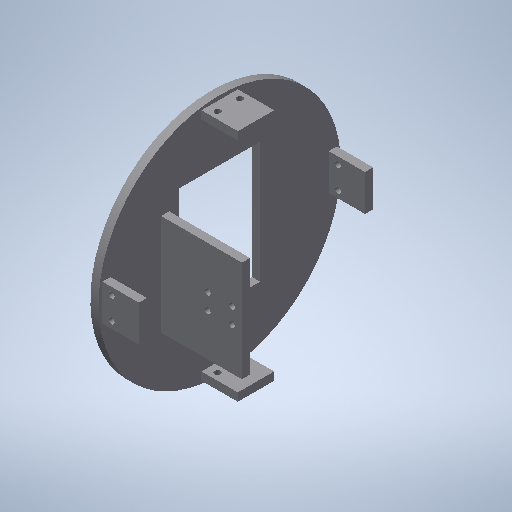
# Autodesk Inventor part: 零件2
Saved by Autodesk Inventor 2025 (Build 290162000, 162)
## iProperties
Created: 2024-03-26
Part Number: 零件2
Material: 常规
Document SubType Name: Modeling
Designer: Administrator
Density: 1 g/cm^3
Appearance: 默认
Author: Administrator
Autodesk Inventor part; units mm, degrees
ref_plane "YZ Plane" through (0, 0, 0) normal (1, 0, 0) x (0, 1, 0)
ref_plane "XZ Plane" through (0, 0, 0) normal (0, 1, 0) x (-1, 0, 0)
ref_plane "XY Plane" through (0, 0, 0) normal (0, 0, 1) x (1, 0, 0)
sketch "草图2" plane through (0, 0, 0) normal (1, 0, 0) x (0, 1, 0)
  arc A0 (-53.1995, 32.7287) -> (-53.1995, 62.7287) centre (4.8952, 47.7287) ccw
  line L0 (4.8952, 17.7287) -> (24.8952, 17.7287)
  line L1 (24.8952, 17.7287) -> (24.8952, 77.7287)
  line L2 (24.8952, 77.7287) -> (-15.1048, 77.7287)
  line L3 (-15.1048, 77.7287) -> (-15.1048, 17.7287)
  line L4 (-15.1048, 17.7287) -> (4.8952, 17.7287)
  arc A1 (-53.1995, 62.7287) -> (-53.1995, 32.7287) centre (4.8952, 47.7287) ccw
  point P0 (0, 0)
  constraints: 10 end point, 4 point on circle, 2 centre point, 1 coincident, 1 collinear, 1 concentric, 1 parallel
extrude "拉伸2" add sketch "草图2" along normal blind 4
sketch "草图3" plane through (4, 4.8952, 47.7287) normal (1, 0, 0) x (0, 0, -1)
  line L0 (-9, 58) -> (9, 58)
  line L1 (9, 58) -> (9, 54)
  line L2 (9, 54) -> (-9, 54)
  line L3 (-9, 54) -> (-9, 58)
  line L4 (0, -74) -> (0, 175)
  line L5 (0, 0) -> (111.1859, 0)
  line L6 (-9, -58) -> (9, -58)
  line L7 (9, -58) -> (9, -54)
  line L8 (9, -54) -> (-9, -54)
  line L9 (-9, -54) -> (-9, -58)
  line L10 (54, 9) -> (58, 9)
  line L11 (58, 9) -> (58, -9)
  line L12 (58, -9) -> (54, -9)
  line L13 (54, -9) -> (54, 9)
  line L14 (-54, 9) -> (-58, 9)
  line L15 (-58, 9) -> (-58, -9)
  line L16 (-58, -9) -> (-54, -9)
  line L17 (-54, -9) -> (-54, 9)
  dimension "d21" = 18
  dimension "d22" = 4
  dimension "d23" = 18
  dimension "d24" = 4
  dimension "d25" = 108
  dimension "d26" = 108
  constraints: 36 end point, 8 symmetric about line, 4 parallel, 3 horizontal, 3 point on line, 2 perpendicular, 1 coincident, 1 vertical, 3 other
  measures "d21" distance of L0.start L0.end
  measures "d22" distance between parallel lines of L2 L0
  measures "d23" distance of L10.end L11.end
  measures "d24" distance between parallel lines of L11 L13
  measures "d25" diameter of L2 L5
  measures "d26" distance between parallel lines of L13 L17
extrude "拉伸3" add sketch "草图3" along normal blind 18
sketch "草图4" plane through (4, -4.1048, -10.2713) normal (0, 0, -1) x (-1, 0, 0)
  line L0 (-4.5, 27) -> (-4.5, -16)
  line L1 (0, 69) -> (0, -51) projected
  line L2 (0, 0) -> (-18, 0) projected
  line L3 (0, 18) -> (-18, 18) projected
  line L4 (2.402, 9) -> (-9.4185, 9) construction
  circle A0 centre (-4.5, 14.5) radius 1.5
  circle A1 centre (-4.5, 3.5) radius 1.5
  point P0 (4, 4.1048)
  point P1 (-2.25, 9)
  dimension "d29" = 4.5
  dimension "d30" = 3
  dimension "d31" = 11
  constraints: 4 end point, 3 point on line, 2 centre point, 1 equal radius, 1 horizontal, 1 vertical, 1 other
  measures "d29" distance between parallel lines of L0 L1
  measures "d30" diameter of A0
  measures "d31" distance of A1.centre A0.centre
extrude "拉伸4" cut sketch "草图4" against normal blind 200 contours A0 L0 | L0 A0 | A1 L0 | L0 A1
sketch "草图6" plane through (4, -53.1048, 38.7287) normal (0, -1, 0) x (1, 0, 0)
  line L0 (4.5, -6) -> (4.5, 26.379)
  line L1 (0, -51) -> (0, 69) projected
  line L2 (0, 18) -> (18, 18) projected
  line L3 (-1.6886, 9) -> (9.3114, 9) construction
  circle A0 centre (4.5, 3.5) radius 1.5
  circle A1 centre (4.5, 14.5) radius 1.5
  point P0 (-4, -38.7287)
  point P1 (2.25, 9)
  dimension "d34" = 4.5
  dimension "d35" = 3
  dimension "d36" = 11
  constraints: 4 end point, 3 point on line, 2 centre point, 1 vertical, 2 other
  measures "d34" distance between parallel lines of L0 L1
  measures "d35" diameter of A0
  measures "d36" distance of A1.centre A0.centre
extrude "拉伸5" cut sketch "草图6" against normal blind 200
sketch "草图7" plane through (4, 4.8952, 47.7287) normal (1, 0, 0) x (0, 0, -1)
  line L0 (-22.6667, -29) -> (27.3333, -29)
  line L1 (27.3333, -29) -> (27.3333, -25)
  line L2 (27.3333, -25) -> (-22.6667, -25)
  line L3 (-22.6667, -25) -> (-22.6667, -29)
  line L4 (30, -20) -> (-30, -20) projected
  line L5 (0, -20) -> (0, -25)
  point P0 (47.7287, -4.8952)
  dimension "d39" = 4
  dimension "d40" = 50
  dimension "d41" = 5
  constraints: 10 end point, 2 parallel, 2 perpendicular, 1 horizontal, 1 midpoint, 1 point on line
  measures "d39" distance between parallel lines of L2 L0
  measures "d40" distance of L1.end L2.end
  measures "d41" distance of L5.start L5.end
extrude "拉伸6" add sketch "草图7" along normal blind 40
sketch "草图8" plane through (4, -24.1048, 20.3953) normal (0, -1, 0) x (1, 0, 0)
  line L0 (40, 0) -> (40, 50) projected
  line L1 (40, 50) -> (40, 25)
  line L2 (40, 25) -> (35, 25)
  line L3 (35, 25) -> (35, 21)
  line L4 (35, 25) -> (35, 29)
  line L5 (35, 25) -> (23, 25)
  line L6 (23, 25) -> (23, 21)
  line L7 (23, 25) -> (23, 29)
  circle A0 centre (35, 21) radius 1.5
  circle A1 centre (35, 29) radius 1.5
  circle A2 centre (23, 29) radius 1.5
  circle A3 centre (23, 21) radius 1.5
  point P0 (-4, -20.3953)
  dimension "d44" = 5
  dimension "d46" = 4
  dimension "d50" = 3
  dimension "d51" = 3
  dimension "d52" = 3
  constraints: 14 end point, 4 centre point, 4 coincident, 3 vertical, 2 perpendicular, 1 horizontal, 1 midpoint
  measures "d44" distance of L1.end L2.end
  measures "d46" distance of L2.end L4.end
  measures "d50" diameter of A1
  measures "d51" diameter of A2
  measures "d52" diameter of A3
extrude "拉伸7" cut sketch "草图8" against normal blind 40
